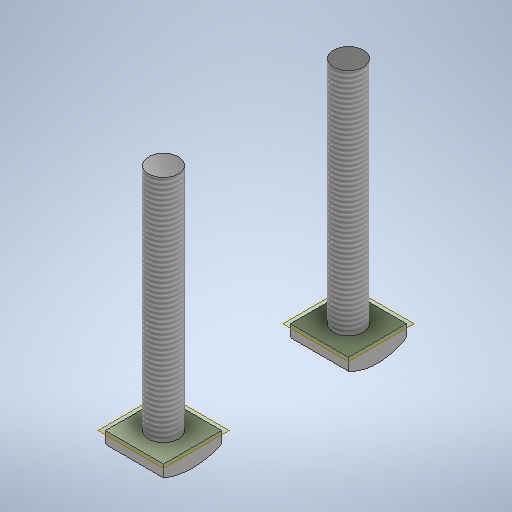
# Autodesk Inventor part: SCREW
Saved by Autodesk Inventor 2025.2 (Build 292293000, 293)
## iProperties
Created: 2025-04-15
Part Number: SCREW
Material: Steel, Mild
Document SubType Name: Modeling
Designer: bless
Density: 7.85 g/cm^3
Appearance: Semi-Polished
Author: bless
Autodesk Inventor part; units mm, degrees
ref_plane "YZ Plane" through (0, 0, 0) normal (1, 0, 0) x (0, 1, 0)
ref_plane "XZ Plane" through (0, 0, 0) normal (0, 1, 0) x (-1, 0, 0)
ref_plane "XY Plane" through (0, 0, 0) normal (0, 0, 1) x (1, 0, 0)
ref_plane "Work Plane1" through (-28.7199, -40.5866, -26.6951) normal (0, -1, 0) x (1, 0, 0)
sketch "Sketch1" plane through (-28.7199, -40.5866, -26.6951) normal (0, -1, 0) x (1, 0, 0)
  line L0 (9.75, 9.75) -> (-9.75, 9.75)
  line L1 (-9.75, 9.75) -> (-9.75, -9.75)
  line L2 (-9.75, -9.75) -> (9.75, -9.75)
  line L3 (9.75, -9.75) -> (9.75, 9.75)
  line L4 (9.75, 9.75) -> (-9.75, -9.75) construction
  line L5 (-9.75, 9.75) -> (9.75, -9.75) construction
  circle A0 centre (0, 0) radius 5
  point P0 (28.7199, 26.6951)
  dimension "d0" = 19.5
  dimension "d1" = 19.5
  dimension "d2" = 10
  constraints: 12 end point, 2 midpoint, 2 parallel, 1 centre point, 1 coincident, 1 horizontal, 1 perpendicular
  measures "d0" distance of L2.end L1.end
  measures "d1" distance of L1.end L0.end
  measures "d2" diameter of A0
extrude "Extrusion1" add sketch "Sketch1" against normal blind 77 contours A0
thread "Thread1" size "M10x1.5" class "6g" standard "ANSI Metric M Profile" length 76
sketch "Sketch2" plane through (-28.7199, -40.5866, -26.6951) normal (0, -1, 0) x (1, 0, 0)
  circle A0 centre (0, 0) radius 5 projected
  line L0 (9.75, 9.75) -> (-9.75, 9.75)
  line L1 (-9.75, 9.75) -> (-9.75, -9.75)
  line L2 (-9.75, -9.75) -> (9.75, -9.75)
  line L3 (9.75, -9.75) -> (9.75, 9.75)
  line L4 (9.75, 9.75) -> (-9.75, -9.75) construction
  line L5 (-9.75, 9.75) -> (9.75, -9.75) construction
  point P0 (28.7199, 26.6951)
  dimension "d7" = 19.5
  dimension "d8" = 19.5
  constraints: 12 end point, 2 midpoint, 2 parallel, 1 horizontal, 1 perpendicular
  measures "d7" distance of L2.end L1.end
  measures "d8" distance of L1.end L0.end
extrude "Extrusion2" add sketch "Sketch2" along normal blind 4.02 contours A0 | L3 L2 L1 L0
sketch "Sketch3" plane through (-18.9699, -40.5866, -16.9451) normal (1, 0, 0) x (0, 0, -1)
  line L0 (19.5, -4.02) -> (0, -4.02) projected
  arc A0 (0, -4.02) -> (19.5, -4.02) centre (9.75, 19.0004) ccw
  point P0 (-16.9451, 40.5866)
  dimension "d11" = 25
  constraints: 2 point on circle, 1 centre point
  measures "d11" radius of A0
extrude "Extrusion3" add sketch "Sketch3" against normal blind 19.5
ref_plane "Work Plane2" through (-28.7159, -40.5866, -88.6951) normal (0, -1, 0) x (1, 0, 0)
sketch "Sketch4" plane through (-28.7159, -40.5866, -88.6951) normal (0, -1, 0) x (1, 0, 0)
  circle A0 centre (0, 0) radius 5 projected
  circle A1 centre (0, 0) radius 5
  line L0 (9.75, 9.75) -> (-9.75, 9.75)
  line L1 (-9.75, 9.75) -> (-9.75, -9.75)
  line L2 (-9.75, -9.75) -> (9.75, -9.75)
  line L3 (9.75, -9.75) -> (9.75, 9.75)
  line L4 (9.75, 9.75) -> (-9.75, -9.75) construction
  line L5 (-9.75, 9.75) -> (9.75, -9.75) construction
  point P0 (28.7159, 88.6951)
  dimension "d14" = 19.5
  dimension "d15" = 19.5
  constraints: 12 end point, 2 midpoint, 2 parallel, 1 centre point, 1 coincident, 1 concentric, 1 horizontal, 1 perpendicular
  measures "d14" distance of L2.end L1.end
  measures "d15" distance of L1.end L0.end
extrude "Extrusion4" add sketch "Sketch4" against normal blind 77 contours A0
sketch "Sketch5" plane through (-28.7159, -40.5866, -88.6951) normal (0, -1, 0) x (1, 0, 0)
  circle A0 centre (0, 0) radius 5 projected
  line L0 (9.75, 9.75) -> (-9.75, 9.75)
  line L1 (-9.75, 9.75) -> (-9.75, -9.75)
  line L2 (-9.75, -9.75) -> (9.75, -9.75)
  line L3 (9.75, -9.75) -> (9.75, 9.75)
  line L4 (9.75, 9.75) -> (-9.75, -9.75) construction
  line L5 (-9.75, 9.75) -> (9.75, -9.75) construction
  point P0 (28.7159, 88.6951)
  dimension "d18" = 19.5
  dimension "d19" = 19.5
  constraints: 12 end point, 2 midpoint, 2 parallel, 1 horizontal, 1 perpendicular
  measures "d18" distance of L2.end L1.end
  measures "d19" distance of L1.end L0.end
extrude "Extrusion5" add sketch "Sketch5" along normal blind 4.02 contours A0 | L3 L2 L1 L0
sketch "Sketch6" plane through (-18.9659, -40.5866, -78.9451) normal (1, 0, 0) x (0, 0, -1)
  line L0 (19.5, -4.02) -> (0, -4.02) projected
  arc A0 (0, -4.02) -> (19.5, -4.02) centre (9.75, 12.8675) ccw
  point P0 (-78.9451, 40.5866)
  dimension "d22" = 19.5
  constraints: 2 point on circle, 1 centre point
  measures "d22" radius of A0
extrude "Extrusion6" add sketch "Sketch6" against normal blind 19.5
thread "Thread2" size "M10x1.5" class "6g" standard "ANSI Metric M Profile" length 76
body "Solid1"
